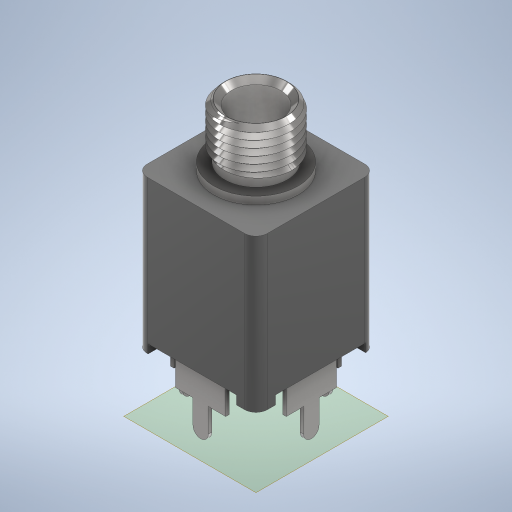
# Autodesk Inventor part: Jack_tht_6-3
Saved by Autodesk Inventor 2023 (Build 270158000, 158)
## iProperties
Created: 2023-04-18
Part Number: Jack_tht_6-3
Material: Generic
Document SubType Name: Modeling
Designer: dvorakj
Density: 1 g/cm^3
Appearance: Default
Author: dvorakj
Autodesk Inventor part; units mm, degrees
ref_plane "YZ Plane" through (0, 0, 0) normal (1, 0, 0) x (0, 1, 0)
ref_plane "XZ Plane" through (0, 0, 0) normal (0, 1, 0) x (-1, 0, 0)
ref_plane "XY Plane" through (0, 0, 0) normal (0, 0, 1) x (1, 0, 0)
sketch "Sketch1" plane through (0, 0, 0) normal (0, 1, 0) x (-1, 0, 0)
  line L0 (15.7, 0) -> (15.7, -11)
  line L1 (15.7, -11) -> (11, -15.7)
  line L2 (11, -15.7) -> (0, -15.7)
  line L3 (0, -15.7) -> (0, 0)
  line L4 (0, 0) -> (15.7, 0)
  dimension "d0" = 15.7
  dimension "d1" = 15.7
  dimension "d2" = 135
  dimension "d3" = 11
  constraints: 10 end point, 3 perpendicular, 1 vertical
  measures "d0" distance of L2.end L3.end
  measures "d1" distance of L3.end L0.start
  measures "d2" angle of L1 L0
  measures "d3" distance of L1.end L2.end
extrude "Extrusion1" add sketch "Sketch1" along normal blind 18.8
sketch "Sketch2" plane through (0, 0, 0) normal (0, -1, 0) x (1, 0, 0)
  line L0 (0, 0) -> (0, -15.7) projected
  line L1 (-15.7, 0) -> (0, 0) projected
  line L2 (-15.7, -11) -> (-15.7, 0) projected
  line L3 (-11, -15.7) -> (-15.7, -11) projected
  line L4 (0, -15.7) -> (-11, -15.7) projected
  line L5 (-11, -15.7) -> (-15.7, -11) projected
  line L6 (-14.941, -11.759) -> (-14.2339, -11.0519)
  line L7 (-14.2339, -11.0519) -> (-11.0519, -14.2339)
  line L8 (-11.0519, -14.2339) -> (-11.759, -14.941)
  line L9 (-11, -15.7) -> (-15.7, -11)
  line L10 (-13.35, -13.35) -> (-12.6429, -12.6429) construction
  line L11 (-15.7, -11) -> (-15.7, 0) projected
  line L12 (-15.7, -3.7) -> (-13, -3.7)
  line L13 (-13, -3.7) -> (-13, -1.71)
  line L14 (-13, -1.71) -> (-14.1, -1.71)
  line L15 (-14.1, -1.71) -> (-14.1, 0)
  line L16 (-15.7, 0) -> (0, 0) projected
  line L17 (0, 0) -> (0, -15.7) projected
  line L18 (0, -2.54) -> (-1.19, -2.54)
  line L19 (-1.19, -2.54) -> (-2.54, -1.19)
  line L20 (-2.54, -1.19) -> (-2.54, 0)
  line L21 (0, -14.35) -> (-2.54, -14.35)
  line L22 (-2.54, -14.35) -> (-2.54, -15.7)
  line L23 (0, -14.35) -> (0, -15.7)
  line L24 (0, -2.54) -> (0, 0)
  line L25 (-2.54, 0) -> (0, 0)
  line L26 (0, -15.7) -> (-11, -15.7) projected
  line L27 (-2.54, -15.7) -> (0, -15.7)
  line L28 (-15.7, -3.7) -> (-15.7, 0)
  line L29 (-14.1, 0) -> (-15.7, 0)
  point P0 (-15.7, -3.7)
  point P1 (-2.54, 0)
  point P2 (0, -14.35)
  point P3 (-14.941, -11.759)
  dimension "d6" = 4.5
  dimension "d7" = 1
  dimension "d8" = 3.7
  dimension "d9" = 1.6
  dimension "d10" = 2.7
  dimension "d11" = 1.71
  dimension "d12" = 2.54
  dimension "d13" = 2.54
  dimension "d14" = 1.35
  dimension "d15" = 1.35
  dimension "d16" = 2.54
  dimension "d17" = 1.35
  constraints: 40 end point, 10 perpendicular, 8 point on line, 5 collinear, 2 horizontal, 2 midpoint, 2 vertical
  measures "d6" distance of L6.end L7.end
  measures "d7" distance of L6.start L6.end
  measures "d8" distance between parallel lines of L1 L12
  measures "d9" distance between parallel lines of L2 L15
  measures "d10" distance between parallel lines of L2 L13
  measures "d11" distance between parallel lines of L1 L14
  measures "d12" distance between parallel lines of L0 L20
  measures "d13" distance between parallel lines of L1 L18
  measures "d14" distance from line of L19.end L18
  measures "d15" distance from line of L20 L18.end
  measures "d16" distance of L21.start L21.end
  measures "d17" distance of L21.end L22.end
extrude "Extrusion2" add sketch "Sketch2" along normal blind 1.14 contours L0 L18 L19 L20 L1 | L0 L4 L22 L21 | L15 L14 L13 L12 L2 L1 | L3 L6 L7 L8
fillet "Fillet1" radius 1.5 5 edges at (0, 8.83, 0) (-15.7, 8.83, 0) (-11, 9.4, -15.7) (-15.7, 9.4, -11) (0, 8.83, -15.7)
sketch "Sketch3" plane through (0, 18.8, 0) normal (0, 1, 0) x (1, 0, 0)
  circle A0 centre (-7.85, 7.85) radius 5.5
  line L0 (0, 1.5) -> (0, 14.2) projected
  line L1 (-14.2, 0) -> (-1.5, 0) projected
  point P0 (0, 0)
  point P1 (0, 7.85)
  point P2 (-7.85, 0)
  dimension "d21" = 11
  constraints: 2 midpoint, 1 centre point, 1 horizontal alignment, 1 vertical alignment
  measures "d21" diameter of A0
extrude "Extrusion3" add sketch "Sketch3" along normal blind 1
sketch "Sketch4" plane through (-7.85, 19.8, -7.85) normal (0, 1, 0) x (1, 0, 0)
  circle A0 centre (0, 0) radius 4.67
  circle A1 centre (0, 0) radius 5.5 projected
  point P0 (7.85, -7.85)
  dimension "d24" = 9.34
  constraints: 1 centre point, 1 coincident
  measures "d24" diameter of A0
extrude "Extrusion4" add sketch "Sketch4" along normal blind 7.14 contours A0
sketch "Sketch5" plane through (-7.85, 26.94, -7.85) normal (0, 1, 0) x (1, 0, 0)
  circle A0 centre (0, 0) radius 3.23
  circle A1 centre (0, 0) radius 4.67 projected
  point P0 (7.85, -7.85)
  dimension "d27" = 6.46
  constraints: 1 centre point, 1 coincident
  measures "d27" diameter of A0
extrude "Extrusion5" cut sketch "Sketch5" against normal through all contours A0
chamfer "Chamfer1" distance 0.7 angle 45 2 edges at (-11.08, 26.94, -7.85) (-12.52, 26.94, -7.85)
ref_plane "Work Plane3" through (-7.85, 18.8, -7.85) normal (0, 0, 1) x (1, 0, 0)
sketch "Sketch6" plane through (-7.85, 18.8, -7.85) normal (0, 0, 1) x (1, 0, 0)
  line L0 (0, 18.8187) -> (0, -7.7615)
  line L1 (-4.67, 1) -> (4.67, 1) projected
  line L2 (4.67, 7.44) -> (-4.67, 7.44) projected
  line L3 (4.67, 1) -> (4.67, 7.44) construction
  line L4 (5.5, 1) -> (-5.5, 1) projected
  line L5 (4.67, 2.35) -> (4.08, 2.35)
  line L6 (4.08, 2.35) -> (4.08, 1)
  line L7 (4.08, 1) -> (4.67, 1)
  line L8 (4.67, 1) -> (4.67, 2.35)
  point P0 (7.85, -18.8)
  point P1 (0, 7.44)
  point P2 (4.67, 1)
  dimension "d37" = 8.16
  dimension "d38" = 1.35
  constraints: 10 end point, 3 point on line, 2 parallel, 1 horizontal, 1 midpoint, 1 perpendicular, 1 vertical
  measures "d37" diameter of L6 L0
  measures "d38" distance between parallel lines of L5 L1
revolve "Revolution1" cut sketch "Sketch6" angle 360 about axis through (-7.85, 37.6187, -7.85) along (0, -1, 0)
sketch "Sketch7" plane through (-7.85, 18.8, -7.85) normal (0, 0, 1) x (1, 0, 0)
  line L0 (4.67, 2.35) -> (-4.67, 2.35) projected
  line L1 (4.67, 7.44) -> (-4.67, 7.44) projected
  line L2 (0, 14.585) -> (0, -6.0348)
  line L3 (4.67, 2.35) -> (4.08, 2.8)
  line L4 (4.08, 2.8) -> (4.67, 3.25)
  line L5 (4.67, 2.35) -> (4.67, 7.44) projected
  line L6 (4.08, 2.35) -> (4.08, 1) construction
  line L7 (4.67, 3.25) -> (4.67, 2.35)
  point P0 (7.85, -18.8)
  point P1 (0, 7.44)
  point P2 (4.67, 2.8)
  dimension "d40" = 0.9
  constraints: 8 end point, 2 midpoint, 2 point on line, 2 vertical, 1 horizontal alignment, 1 vertical alignment
  measures "d40" distance of L0.start L4.end
coil "Coil1" sketch "Sketch7" operation cut axis through (-7.85, 33.385, -7.85) along (0, 1, 0) pitch 0.9 turns 6 hand right contours L3 L4 L5
coil "Coil2" sketch "Sketch7" operation cut axis through (-7.85, 33.385, -7.85) along (0, -1, 0) pitch 0.9 turns 1 hand right contours L3 L4 L5
sketch "Sketch8" plane through (0, 0, 0) normal (0, -1, 0) x (1, 0, 0)
  circle A0 centre (-7.85, -7.85) radius 3.23 projected
  arc A1 (-0.0075, -14.35) -> (0, -14.2) centre (-1.5, -14.2) ccw projected
  line L0 (0, -2.54) -> (0, -14.2) projected
  line L1 (0, -2.54) -> (-1.19, -2.54) projected
  line L2 (-1.19, -2.54) -> (-2.54, -1.19) projected
  line L3 (-2.54, -1.19) -> (-2.54, 0) projected
  line L4 (-14.1, 0) -> (-2.54, 0) projected
  line L5 (-14.1, 0) -> (-14.1, -1.71) projected
  line L6 (-14.1, -1.71) -> (-13, -1.71) projected
  line L7 (-13, -1.71) -> (-13, -3.7) projected
  line L8 (-13, -3.7) -> (-15.7, -3.7) projected
  line L9 (-15.7, -10.3787) -> (-15.7, -3.7) projected
  arc A2 (-15.7, -10.3787) -> (-15.2607, -11.4393) centre (-14.2, -10.3787) ccw projected
  line L10 (-14.941, -11.759) -> (-14.2339, -11.0519) projected
  line L11 (-14.2339, -11.0519) -> (-11.0519, -14.2339) projected
  line L12 (-11.0519, -14.2339) -> (-11.759, -14.941) projected
  arc A3 (-11.4393, -15.2607) -> (-10.3787, -15.7) centre (-10.3787, -14.2) ccw projected
  line L13 (-2.54, -15.7) -> (-10.3787, -15.7) projected
  line L14 (-2.54, -15.7) -> (-2.54, -14.35) projected
  line L15 (-2.54, -14.35) -> (-0.0075, -14.35) projected
  line L16 (-1.22, -11.73) -> (-1.68, -11.73)
  line L17 (-1.68, -11.73) -> (-1.68, -5.17)
  line L18 (-1.68, -5.17) -> (-1.22, -5.17)
  line L19 (-1.22, -5.17) -> (-1.22, -11.73)
  line L20 (-5.17, -1.68) -> (-11.73, -1.68)
  line L21 (-11.73, -1.68) -> (-11.73, -1.22)
  line L22 (-11.73, -1.22) -> (-5.17, -1.22)
  line L23 (-5.17, -1.22) -> (-5.17, -1.68)
  line L24 (-14.48, -3.315) -> (-14.02, -3.315)
  line L25 (-14.02, -3.315) -> (-14.02, -7.585)
  line L26 (-14.02, -7.585) -> (-14.48, -7.585)
  line L27 (-14.48, -7.585) -> (-14.48, -3.315)
  line L28 (-3.315, -14.48) -> (-7.585, -14.48)
  line L29 (-7.585, -14.48) -> (-7.585, -14.02)
  line L30 (-7.585, -14.02) -> (-3.315, -14.02)
  line L31 (-3.315, -14.02) -> (-3.315, -14.48)
  line L32 (-11.173, -14.1923) -> (-14.1923, -11.173)
  line L33 (-14.1923, -11.173) -> (-13.867, -10.8477)
  line L34 (-13.867, -10.8477) -> (-10.8477, -13.867)
  line L35 (-10.8477, -13.867) -> (-11.173, -14.1923)
  line L36 (-14.941, -11.759) -> (-11.759, -14.941) projected
  line L37 (-13.35, -13.35) -> (-12.6826, -12.6826) construction
  line L38 (-12.3574, -12.3574) -> (-12.6826, -12.6826) construction
  line L39 (-14.941, -11.759) -> (-15.2607, -11.4393) projected
  line L40 (-11.4393, -15.2607) -> (-11.759, -14.941) projected
  point P0 (0, 0)
  point P1 (-14.5607, -11.4393)
  point P2 (-11.4393, -14.5607)
  point P3 (-14.25, -7.585)
  point P4 (-1.45, -5.17)
  point P5 (-11.73, -1.45)
  point P6 (-7.585, -14.25)
  point P7 (-14.48, -5.45)
  point P8 (-12.52, -12.52)
  point P9 (-8.45, -1.22)
  point P10 (-1.68, -8.45)
  point P11 (-5.45, -14.02)
  dimension "d57" = 0.46
  dimension "d63" = 0.46
  dimension "d64" = 0.46
  dimension "d65" = 0.46
  dimension "d66" = 0.46
  dimension "d67" = 6.56
  dimension "d68" = 6.56
  dimension "d69" = 4.27
  dimension "d70" = 4.27
  dimension "d71" = 4.27
  dimension "d86" = 6.4
  dimension "d87" = 6.4
  dimension "d88" = 6.4
  dimension "d89" = 6.4
  dimension "d90" = 2.4
  dimension "d91" = 4.67
  dimension "d104" = 2.4
  dimension "d105" = 0.6
  dimension "d106" = 0.6
  constraints: 44 end point, 11 midpoint, 8 parallel, 8 perpendicular, 4 horizontal, 3 other
  measures "d57" distance of L28.end L29.end
  measures "d63" distance of L16.start L16.end
  measures "d64" distance of L25.end L26.end
  measures "d65" distance of L32.end L33.end
  measures "d66" distance of L20.end L21.end
  measures "d67" distance between parallel lines of L18 L16
  measures "d68" distance from line of L21.end L23
  measures "d69" distance between parallel lines of L26 L24
  measures "d70" distance between parallel lines of L35 L33
  measures "d71" distance between parallel lines of L31 L29
  measures "d86" horizontal distance of A0.centre point (-1.45, -5.17)
  measures "d87" horizontal distance of point (-14.25, -7.585) A0.centre
  measures "d88" vertical distance of A0.centre point (-11.73, -1.45)
  measures "d89" vertical distance of point (-7.585, -14.25) A0.centre
  measures "d90" vertical distance of A0.centre point (-14.48, -5.45)
  measures "d91" horizontal distance of point (-12.52, -12.52) A0.centre
  measures "d104" horizontal distance of A0.centre point (-5.45, -14.02)
  measures "d105" horizontal distance of point (-8.45, -1.22) A0.centre
  measures "d106" vertical distance of point (-1.68, -8.45) A0.centre
extrude "Extrusion6" add sketch "Sketch8" along normal blind 4.37 contours L35 L32 L33 L11 | L11 L33 L34 L35 | L25 L26 L27 L8 | L8 L27 L24 L25 | L16 L17 L18 L19 | L20 L21 L22 L23 | L28 L29 L30 L31
sketch "Sketch9" plane through (0, -4.37, 0) normal (0, -1, 0) x (1, 0, 0)
  line L0 (-5.17, -1.22) -> (-11.73, -1.22) projected
  line L1 (-11.73, -1.22) -> (-11.73, -1.68) projected
  line L2 (-11.73, -1.68) -> (-5.17, -1.68) projected
  line L3 (-5.17, -1.68) -> (-5.17, -1.22) projected
  line L4 (-14.48, -3.315) -> (-14.48, -7.585) projected
  line L5 (-14.48, -7.585) -> (-14.02, -7.585) projected
  line L6 (-14.02, -7.585) -> (-14.02, -3.315) projected
  line L7 (-14.02, -3.315) -> (-14.48, -3.315) projected
  line L8 (-10.8477, -13.867) -> (-13.867, -10.8477) projected
  line L9 (-13.867, -10.8477) -> (-14.1923, -11.173) projected
  line L10 (-14.1923, -11.173) -> (-11.173, -14.1923) projected
  line L11 (-11.173, -14.1923) -> (-10.8477, -13.867) projected
  line L12 (-3.315, -14.02) -> (-7.585, -14.02) projected
  line L13 (-7.585, -14.02) -> (-7.585, -14.48) projected
  line L14 (-7.585, -14.48) -> (-3.315, -14.48) projected
  line L15 (-3.315, -14.48) -> (-3.315, -14.02) projected
  line L16 (-1.22, -5.17) -> (-1.68, -5.17) projected
  line L17 (-1.68, -5.17) -> (-1.68, -11.73) projected
  line L18 (-1.68, -11.73) -> (-1.22, -11.73) projected
  line L19 (-1.22, -11.73) -> (-1.22, -5.17) projected
  line L20 (-9.45, -1.22) -> (-7.45, -1.22)
  line L21 (-7.45, -1.22) -> (-7.45, -1.68)
  line L22 (-7.45, -1.68) -> (-9.45, -1.68)
  line L23 (-9.45, -1.68) -> (-9.45, -1.22)
  line L24 (-1.68, -7.45) -> (-1.22, -7.45)
  line L25 (-1.22, -7.45) -> (-1.22, -9.45)
  line L26 (-1.22, -9.45) -> (-1.68, -9.45)
  line L27 (-1.68, -9.45) -> (-1.68, -7.45)
  line L28 (-6.45, -14.02) -> (-4.45, -14.02)
  line L29 (-4.45, -14.02) -> (-4.45, -14.48)
  line L30 (-4.45, -14.48) -> (-6.45, -14.48)
  line L31 (-6.45, -14.48) -> (-6.45, -14.02)
  line L32 (-14.48, -7.585) -> (-14.48, -3.7) projected
  line L33 (-14.02, -3.7) -> (-14.02, -7.585) projected
  line L34 (-14.48, -4.45) -> (-14.02, -4.45)
  line L35 (-14.02, -4.45) -> (-14.02, -6.45)
  line L36 (-14.02, -6.45) -> (-14.48, -6.45)
  line L37 (-14.48, -6.45) -> (-14.48, -4.45)
  line L38 (-13.3897, -11.9755) -> (-13.0645, -11.6503)
  line L39 (-13.0645, -11.6503) -> (-11.6503, -13.0645)
  line L40 (-11.6503, -13.0645) -> (-11.9755, -13.3897)
  line L41 (-11.9755, -13.3897) -> (-13.3897, -11.9755)
  point P0 (0, 0)
  point P1 (-8.45, -1.68)
  point P2 (-1.22, -8.45)
  point P3 (-14.02, -5.45)
  point P4 (-14.02, -5.45)
  point P5 (-14.48, -5.45)
  point P6 (-14.48, -5.45)
  point P7 (-5.45, -14.48)
  point P8 (-1.68, -9.45)
  point P9 (-1.22, -7.45)
  point P10 (-14.02, -6.45)
  point P11 (-14.02, -4.45)
  point P12 (-9.45, -1.68)
  point P13 (-7.45, -1.22)
  point P14 (-12.3574, -12.3574)
  dimension "d78" = 2
  dimension "d79" = 2
  dimension "d80" = 2
  dimension "d81" = 2
  dimension "d92" = 2
  constraints: 40 end point, 12 point on line, 11 midpoint, 8 parallel, 6 perpendicular, 4 horizontal, 2 coincident, 1 collinear
  measures "d78" distance of L21.end L22.end
  measures "d79" distance of L24.end L25.end
  measures "d80" distance of L29.end L30.end
  measures "d81" distance of L34.end L35.end
  measures "d92" distance between parallel lines of L38 L40
extrude "Extrusion7" add sketch "Sketch9" along normal blind 8.51 from surface at -4.37 contours L21 L2 L23 L0 | L34 L6 L36 L4 | L40 L10 L38 L8 | L29 L14 L31 L12 | L19 L26 L17 L24
fillet "Fillet3" radius 1 10 edges at (-11.8129, -8.51, -13.2271) (-13.2271, -8.51, -11.8129) (-6.45, -8.51, -14.25) (-4.45, -8.51, -14.25) (-1.45, -8.51, -7.45) (-1.45, -8.51, -9.45) (-9.45, -8.51, -1.45) (-7.45, -8.51, -1.45) (-14.25, -8.51, -4.45) (-14.25, -8.51, -6.45)
ref_plane "Work Plane5" through (0, -9, 0) normal (0, -1, 0) x (1, 0, 0)
equation "\"d1\" = d0"
equation "\"d63\" = d57"
equation "\"d64\" = d57"
equation "\"d65\" = d57"
equation "\"d66\" = d65"
equation "\"d70\" = d69"
equation "\"d71\" = d70"
body "Solid1"
